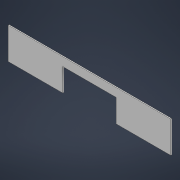
# Autodesk Inventor part: panelFront
Saved by Autodesk Inventor 2021 (Build 250183000, 183)
## iProperties
Created: 2021-11-24
Part Number: panelFront
Material: Generic
Document SubType Name: Modeling
Designer: jo_ki
Density: 1 g/cm^3
Appearance: Default
Author: jo_ki
Autodesk Inventor part; units mm, degrees
ref_plane "YZ Plane" through (0, 0, 0) normal (1, 0, 0) x (0, 1, 0)
ref_plane "XZ Plane" through (0, 0, 0) normal (0, 1, 0) x (-1, 0, 0)
ref_plane "XY Plane" through (0, 0, 0) normal (0, 0, 1) x (1, 0, 0)
sketch "Sketch1" plane through (0, 0, 0) normal (0, 0, 1) x (1, 0, 0)
  line L0 (-340, -66) -> (340, -66)
  line L1 (340, -66) -> (340, 66)
  line L2 (340, 66) -> (-340, 66)
  line L3 (-340, 66) -> (-340, -66)
  line L4 (-340, -66) -> (340, 66) construction
  line L5 (340, -66) -> (-340, 66) construction
  line L6 (-112, -66) -> (112, -66)
  line L7 (112, -66) -> (112, 30)
  line L8 (112, 30) -> (-112, 30)
  line L9 (-112, 30) -> (-112, -66)
  line L10 (-112, -66) -> (112, 30) construction
  line L11 (112, -66) -> (-112, 30) construction
  point P0 (0, 0)
  point P1 (0, -18)
  point P2 (0, 0)
  point P3 (0, -18)
  dimension "d1" = 680
  dimension "d2" = 132
  dimension "d3" = 96
  dimension "d4" = 224
  constraints: 24 end point, 6 midpoint, 4 parallel, 2 horizontal, 2 perpendicular, 1 collinear, 1 vertical alignment
  measures "d1" distance between parallel lines of L3 L1
  measures "d2" distance of L0.end L1.end
  measures "d3" distance of L6.end L7.end
  measures "d4" distance of L7.end L8.end
derived "Mastersketch.ipt"
extrude "Extrusion1" add sketch "Sketch1" along normal mid plane 4 contours L3 L2 L1 L0 L7 L8 L9
equation "\"d1\" = feet_widthCenter - profile_width"
equation "\"d2\" = glass_thickness + playAreaWall_height - goalPanel_thickness"
equation "\"d3\" = goal_height"
equation "\"d4\" = goal_width"
equation "\"d5\" = goalPanel_thickness"
equation "\"feet_widthCenter\" = 720"
equation "\"profile_width\" = 40"
equation "\"glass_thickness\" = 6"
equation "\"playAreaWall_height\" = 130"
equation "\"goalPanel_thickness\" = 4"
equation "\"goal_height\" = 96"
equation "\"goal_width\" = 224"
body "Solid1"
